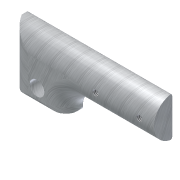
# Autodesk Inventor part: FE-00027
Saved by Autodesk Inventor 2012 (Build 160160000, 160)
## iProperties
Created: 2008-05-25
Part Number: FE-00027
Document SubType Name: Modeling
Designer: firstuser
Density: 1 g/cm^3
Mass: 63.3964 g
Surface Area: 142.366 cm^2
Volume: 63.3964 cm^3
Material: Default
Author: firstuser
Autodesk Inventor part; units mm, degrees
note: some values were not read from the file. Chosen so that the rebuilt part matches the saved one: edges of "Fillet1".
ref_plane "YZ Plane" through (0, 0, 0) normal (1, 0, 0) x (0, 1, 0)
ref_plane "XZ Plane" through (0, 0, 0) normal (0, 1, 0) x (-1, 0, 0)
ref_plane "XY Plane" through (0, 0, 0) normal (0, 0, 1) x (1, 0, 0)
sketch "Sketch1" plane through (0, 0, 0) normal (0, 0, 1) x (1, 0, 0)
  line L0 (0, -4.7625) -> (0, -55.5625)
  line L1 (0, -55.5625) -> (50.8, -55.5625)
  line L2 (50.8, -55.5625) -> (50.8, -50.8)
  line L3 (61.9125, -39.6875) -> (127, -39.6875)
  line L4 (127, -39.6875) -> (127, -4.7625)
  line L5 (127, -4.7625) -> (0, -4.7625)
  arc A0 (61.9125, -39.6875) -> (50.8, -50.8) centre (61.9125, -50.8) ccw
  point P0 (0, -39.6875)
  point P1 (50.8, -39.6875)
  dimension "d0" = 50.8
  dimension "d1" = 34.925
  dimension "d2" = 50.8
  dimension "d3" = 127
  dimension "d8" = 11.1125
  constraints: 12 end point, 4 parallel, 3 point on line, 2 point on circle, 2 tangent, 1 centre point, 1 perpendicular, 1 vertical
  measures "d0" distance of L0.start L0.end
  measures "d1" distance of L3.end L4.end
  measures "d2" distance of L0.end L1.end
  measures "d3" distance of L4.end L0.start
  measures "d8" radius of A0
extrude "Extrusion1" add sketch "Sketch1" along normal blind 19.05
fillet "Fillet1" radius 17.4625 5 edges at (63.5, -4.7625, 19.05) (94.4563, -39.6875, 19.05) (0, -30.1625, 19.05) (54.0548, -42.9423, 19.05) (50.8, -53.1812, 19.05)
sketch "Sketch2" plane through (127, -39.6875, 0) normal (1, 0, 0) x (0, 0, -1)
  line L0 (0, 34.925) -> (0, 0) projected
  line L1 (0, -47.625) -> (-3.175, -47.625)
  line L2 (-3.175, -47.625) -> (-3.175, 155.575)
  line L3 (-3.175, 155.575) -> (0, 155.575)
  line L4 (0, 155.575) -> (0, -47.625)
  dimension "d11" = 3.175
  dimension "d12" = 203.2
  constraints: 8 end point, 2 parallel, 1 collinear, 1 horizontal, 1 perpendicular
  measures "d11" distance of L1.start L1.end
  measures "d12" distance of L1.end L2.end
extrude "Extrusion2" cut sketch "Sketch2" against normal mid plane 1066.8
hole "Hole1" at (114.3, -22.2973, 3.175) direction (0, 0, 1) diameter 4.9784 end through all thread size "1/4-20 UNC" class "2B" standard "ANSI Unified Screw Threads"
pattern_linear "Rectangular Pattern1" count 2 spacing 38.1 along (-1, 0, 0) of "Hole1"
hole "Hole2" at (25.4, -43.9801, 3.175) direction (0, 0, 1) diameter 12.7 end through all
sketch "Sketch3" plane through (0, 0, 0) normal (1, 0, 0) x (0, 1, 0)
  line L0 (-55.5625, 19.05) -> (-55.5625, 3.175) projected
  line L1 (-55.5625, 3.175) -> (-55.5625, 19.05) projected
  line L2 (-22.225, 19.05) -> (-50.8, 19.05) projected
  line L3 (-55.5625, 19.05) -> (-22.225, 19.05) projected
  line L4 (-50.8, 19.05) -> (-55.5625, 19.05) projected
  line L5 (-50.3301, 19.05) -> (-37.6301, 19.05) projected
  line L6 (-37.6301, 3.175) -> (-50.3301, 3.175) projected
  line L7 (-19.8081, 3.175) -> (-24.7865, 3.175) projected
  line L8 (-19.8081, 3.175) -> (-24.7865, 3.175) projected
  line L9 (-4.8348, 3.175) -> (-55.5625, 3.175) projected
  line L10 (-39.6152, 3.175) -> (-4.8348, 3.175) projected
  line L11 (-50.8, 3.175) -> (-39.6152, 3.175) projected
  line L12 (-55.5625, 3.175) -> (-50.8, 3.175) projected
  arc A0 (-52.3875, 19.05) -> (-55.5625, 15.875) centre (-52.3875, 15.875) ccw
  arc A1 (-55.5625, 6.35) -> (-52.3875, 3.175) centre (-52.3875, 6.35) ccw
  line L13 (-52.3875, 19.05) -> (-55.5625, 19.05)
  line L14 (-55.5625, 19.05) -> (-55.5625, 15.875)
  line L15 (-55.5625, 6.35) -> (-55.5625, 3.175)
  line L16 (-55.5625, 3.175) -> (-52.3875, 3.175)
  dimension "d39" = 3.175
  constraints: 8 end point, 6 coincident, 6 tangent, 4 point on circle, 4 point on line, 2 centre point, 2 perpendicular, 1 equal radius
  measures "d39" radius of A0
extrude "Extrusion3" cut sketch "Sketch3" along normal blind 508
sketch "Sketch4" plane through (127, -22.225, 1.5875) normal (1, 0, 0) x (0, 0, -1)
  line L0 (-1.5875, -17.3902) -> (-1.5875, 17.3902) projected
  arc A0 (-1.5875, 17.3902) -> (-1.5875, -17.3902) centre (0, 0) ccw projected
  arc A1 (-1.5875, 15.5543) -> (-3.4925, 17.1097) centre (-3.175, 15.5543) ccw
  arc A2 (-3.4925, -17.1097) -> (-1.5875, -15.5543) centre (-3.175, -15.5543) ccw
  line L1 (-1.5875, 15.5543) -> (0, 15.5543)
  line L2 (0, 15.5543) -> (0, 19.05)
  line L3 (0, 19.05) -> (-3.175, 19.05)
  line L4 (-3.175, 19.05) -> (-3.4925, 17.1097)
  line L5 (-1.5875, -15.5543) -> (0, -15.5543)
  line L6 (0, -15.5543) -> (0, -19.05)
  line L7 (0, -19.05) -> (-3.175, -19.05)
  line L8 (-3.175, -19.05) -> (-3.4925, -17.1097)
  dimension "d42" = 1.5875
  constraints: 16 end point, 6 point on circle, 4 tangent, 2 centre point, 2 perpendicular, 2 point on line, 1 equal radius, 1 parallel
  measures "d42" radius of A2
sketch "Sketch5" plane through (127, -39.6152, 3.175) normal (0, 0, -1) x (-1, 0, 0)
  line L0 (126.9277, 34.7804) -> (126.9277, -12.7723) projected
  arc A0 (76.2723, -11.1848) -> (65.0875, 0) centre (65.0875, -11.1848) ccw projected
  line L1 (0, 34.7804) -> (126.9277, 34.7804)
  line L2 (126.9277, 34.7804) -> (126.9277, -25.4)
  line L3 (0, 0) -> (65.0875, 0)
  line L4 (76.2723, -11.1848) -> (76.2723, -28.575)
  arc A1 (76.2723, -11.1848) -> (65.0875, 0) centre (65.0875, -11.1848) ccw
  constraints: 8 end point, 2 perpendicular, 2 point on circle, 2 tangent, 1 centre point, 1 concentric, 1 point on line
sweep "Sweep1" cut profiles "Sketch4" path "Sketch5" path curves L1 L2 contours A1 A0 L0 | L0 A0 L4 L3 L2 L1
sweep "Sweep2" cut profiles "Sketch4" path "Sketch5" path curves L3 A1 L4 contours A0 A2 L0 | L0 L5 L6 L7 L8 A0
sketch "Sketch6" plane through (127, -6.6707, 3.175) normal (0, 0, -1) x (-1, 0, 0)
  line L0 (0, 1.5554) -> (126.6472, 1.5554) projected
  line L1 (126.6472, 1.5554) -> (126.6472, -48.6267) projected
  line L2 (76.862, -48.8918) -> (126.338, -48.8918) projected
  line L3 (76.5528, -48.6267) -> (76.5528, -44.1293) projected
  arc A0 (76.5528, -45.7168) -> (79.7278, -48.8918) centre (79.7278, -45.7168) ccw
  arc A1 (123.4722, -48.8918) -> (126.6472, -45.7168) centre (123.4722, -45.7168) ccw
  arc A2 (126.6472, -1.6196) -> (123.4722, 1.5554) centre (123.4722, -1.6196) ccw
  line L4 (76.5528, -45.7168) -> (72.1108, -45.7168)
  line L5 (72.1108, -45.7168) -> (71.4375, -52.3875)
  line L6 (71.4375, -52.3875) -> (79.375, -52.3875)
  line L7 (79.375, -52.3875) -> (79.7278, -48.8918)
  line L8 (123.4722, -48.8918) -> (123.4722, -52.3875)
  line L9 (123.4722, -52.3875) -> (130.175, -52.3875)
  line L10 (130.175, -52.3875) -> (130.175, -45.7168)
  line L11 (130.175, -45.7168) -> (126.6472, -45.7168)
  line L12 (123.4722, 1.5554) -> (123.4722, 4.7625)
  line L13 (123.4722, 4.7625) -> (128.8197, 4.2228)
  line L14 (128.8197, 4.2228) -> (128.8197, -1.6196)
  line L15 (128.8197, -1.6196) -> (126.6472, -1.6196)
  dimension "d45" = 6.35
  constraints: 24 end point, 6 perpendicular, 6 point on circle, 6 point on line, 6 tangent, 5 parallel, 3 centre point, 2 equal radius
  measures "d45" diameter of A0
extrude "Extrusion4" cut sketch "Sketch6" against normal blind 508
body "Solid1"
